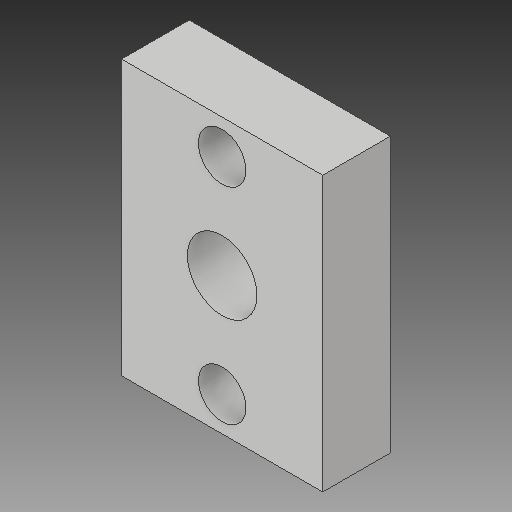
# Autodesk Inventor part: lift top
Saved by Autodesk Inventor 2019 (Build 230136000, 136)
## iProperties
Created: 2018-10-16
Part Number: lift top
Material: Generic
Document SubType Name: Modeling
Designer: User
Density: 1 g/cm^3
Appearance: Default
Author: User
Autodesk Inventor part; units mm, degrees
ref_plane "YZ Plane" through (0, 0, 0) normal (1, 0, 0) x (0, 1, 0)
ref_plane "XZ Plane" through (0, 0, 0) normal (0, 1, 0) x (-1, 0, 0)
ref_plane "XY Plane" through (0, 0, 0) normal (0, 0, 1) x (1, 0, 0)
sketch "Sketch1" plane through (0, 0, 0) normal (0, 0, 1) x (1, 0, 0)
  line L0 (0, 0) -> (27.94, 0)
  line L1 (27.94, 0) -> (27.94, 38.1)
  line L2 (27.94, 38.1) -> (0, 38.1)
  line L3 (0, 38.1) -> (0, 0)
  dimension "d0" = 27.94
  dimension "d1" = 38.1
  constraints: 8 end point, 2 parallel, 1 horizontal, 1 perpendicular
  measures "d0" distance of L2.end L1.end
  measures "d1" distance of L1.end L0.end
extrude "Extrusion1" add sketch "Sketch1" along normal blind 9.398
sketch "Sketch2" plane through (0, 0, 9.398) normal (0, 0, 1) x (1, 0, 0)
  line L0 (0, 0) -> (27.94, 0) projected
  line L1 (27.94, 0) -> (27.94, 38.1) projected
  line L2 (27.94, 38.1) -> (0, 38.1) projected
  line L3 (0, 38.1) -> (0, 0) projected
  point P0 (13.97, 33.3375)
  point P1 (13.97, 4.7625)
  dimension "d4" = 28.575
  dimension "d5" = 38.1
  dimension "d6" = 4.7625
  dimension "d7" = 27.94
  dimension "d8" = 13.97
  dimension "d9" = 13.97
  measures "d4" distance of point (13.97, 4.762) point (13.97, 33.337)
  measures "d5" distance of L2.end L0.start
  measures "d6" distance from line of point (13.97, 4.762) L0
  measures "d7" distance of L1.end L2.end
  measures "d8" distance from line of L3 point (13.97, 33.337)
  measures "d9" distance from line of L3 point (13.97, 4.762)
hole "Hole1" at (13.97, 33.3375, 9.398) at (13.97, 4.7625, 9.398) direction (0, 0, -1) diameter 6.604 depth 10.9728 tip angle 118
sketch "Sketch3" plane through (0, 0, 9.398) normal (0, 0, 1) x (1, 0, 0)
  circle A0 centre (13.97, 33.3375) radius 3.302 projected
  circle A1 centre (13.97, 4.7625) radius 3.302 projected
  line L0 (0, 0) -> (27.94, 0) projected
  line L1 (27.94, 0) -> (27.94, 38.1) projected
  line L2 (27.94, 38.1) -> (0, 38.1) projected
  line L3 (0, 38.1) -> (0, 0) projected
  point P0 (13.97, 19.05)
  dimension "d17" = 27.94
  dimension "d18" = 38.1
  dimension "d19" = 13.97
  dimension "d20" = 19.05
  measures "d17" distance of L1.end L2.end
  measures "d18" distance of L2.end L0.start
  measures "d19" distance from line of L3 point (13.97, 19.05)
  measures "d20" distance from line of L2 point (13.97, 19.05)
hole "Hole2" at (13.97, 19.05, 9.398) direction (0, 0, -1) diameter 9.652 depth 10.9728 tip angle 118
equation "\"d6\" = -0.5 * d4 + 0.5 * d5"
equation "\"d8\" = 0.5 * d7"
equation "\"d9\" = d8"
equation "\"d19\" = 0.5 * d17"
equation "\"d20\" = 0.5 * d18"
body "Solid1"
